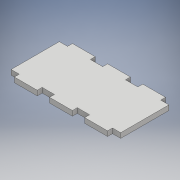
# Autodesk Inventor part: base4
Saved by Autodesk Inventor 2018 (Build 220112000, 112)
## iProperties
Created: 2020-03-10
Part Number: base4
Material: Genérico
Document SubType Name: Modeling
Designer: sala.ceri
Density: 1 g/cm^3
Appearance: Valor por defecto
Author: sala.ceri
Autodesk Inventor part; units mm, degrees
ref_plane "YZ Plane" through (0, 0, 0) normal (1, 0, 0) x (0, 1, 0)
ref_plane "XZ Plane" through (0, 0, 0) normal (0, 1, 0) x (-1, 0, 0)
ref_plane "XY Plane" through (0, 0, 0) normal (0, 0, 1) x (1, 0, 0)
sketch "Boceto1" plane through (0, 0, 0) normal (0, 1, 0) x (-1, 0, 0)
  circle A0 centre (28.5, 0) radius 1.5
  circle A1 centre (28.5, -8) radius 1.5
  circle A2 centre (28.5, 8) radius 1.5
  circle A3 centre (36.5, 0) radius 1.5
  circle A4 centre (20.5, 0) radius 1.5
  circle A5 centre (28.5, 0) radius 47.5
  line L0 (57, 33) -> (43, 33)
  line L1 (43, 33) -> (43, 30)
  line L2 (35.5, 30) -> (35.5, 33)
  line L3 (35.5, 33) -> (21.5, 33)
  line L4 (21.5, 33) -> (21.5, 30)
  line L5 (14, 30) -> (14, 33)
  line L6 (14, 33) -> (0, 33)
  line L7 (43, 30) -> (57, 30)
  line L8 (21.5, 30) -> (35.5, 30)
  line L9 (14, 30) -> (0, 30)
  line L10 (0, 30) -> (0, 33)
  line L11 (57, 33) -> (57, 30)
  line L12 (35.5, -30) -> (35.5, -33)
  line L13 (21.5, -30) -> (35.5, -30)
  line L14 (35.5, -33) -> (21.5, -33)
  line L15 (21.5, -33) -> (21.5, -30)
  line L16 (57, -33) -> (43, -33)
  line L17 (43, -33) -> (43, -30)
  line L18 (43, -30) -> (57, -30)
  line L19 (14, -30) -> (14, -33)
  line L20 (14, -30) -> (0, -30)
  line L21 (14, -33) -> (0, -33)
  line L22 (0, -30) -> (0, -33)
  line L23 (57, -33) -> (57, -30)
  constraints: 48 end point, 10 point on line, 6 centre point, 1 coincident, 1 vertical
extrude "Extrusión1" add sketch "Boceto1" along normal blind 3
sketch "Boceto2" plane through (-28.5, 0, 0) normal (0, -1, 0) x (1, 0, 0)
  circle A0 centre (0, 0) radius 3.5
  point P0 (28.5, 0)
  dimension "d23" = 7
  constraints: 1 centre point
  measures "d23" diameter of A0
extrude "Extrusión2" cut sketch "Boceto2" against normal blind 10
sketch "Boceto3" plane through (-28.5, 0, 0) normal (0, -1, 0) x (1, 0, 0)
  circle A0 centre (0, 0) radius 4.5
  point P0 (28.5, 0)
  dimension "d26" = 9
  constraints: 1 centre point
  measures "d26" diameter of A0
extrude "Extrusión3" cut sketch "Boceto3" against normal blind 10
sketch "Boceto4" plane through (-28.5, 0, 0) normal (0, -1, 0) x (1, 0, 0)
  circle A0 centre (0, 0) radius 4.5 projected
  arc A1 (-38.8091, 27.388) -> (38.8091, 27.388) centre (0, 0) ccw
  line L0 (-28.5, 30) -> (-28.5, 33) projected
  line L1 (-28.5, 30) -> (-28.5, 33)
  line L2 (-28.5, 33) -> (28.5, 33)
  line L3 (28.5, 33) -> (28.5, 30)
  line L4 (-14.5, 30) -> (-28.5, 30) projected
  line L5 (28.5, 30) -> (-28.5, 30)
  line L6 (-28.5, 33) -> (-31.5138, 33)
  line L7 (-31.5138, 33) -> (-31.5138, 30)
  line L8 (-31.5138, 30) -> (-28.5, 30)
  circle A2 centre (0, 0) radius 47.5 projected
  line L9 (38.8091, 27.388) -> (-38.8091, 27.388)
  point P0 (28.5, 0)
  constraints: 16 end point, 4 perpendicular, 4 point on circle, 2 horizontal, 1 centre point, 1 coincident, 1 collinear, 1 vertical
extrude "Extrusión4" cut sketch "Boceto4" against normal blind 10 contours L9 A1
sketch "Boceto5" plane through (0, 0, 0) normal (0, -1, 0) x (1, 0, 0)
  arc A0 (10.3091, 27.388) -> (-67.3091, 27.388) centre (-28.5, 0) ccw projected
  arc A1 (10.3091, 27.388) -> (-67.3091, 27.388) centre (-28.5, 0) ccw
  line L0 (-57, 19.347) -> (-43, 19.347)
  line L1 (0, 19.347) -> (-14, 19.347)
  line L2 (-14, 19.347) -> (-14, 16.347)
  line L3 (-21.5, 16.347) -> (-35.5, 16.347)
  line L4 (-43, 16.347) -> (-57, 16.347)
  line L5 (-57, 19.347) -> (-57, 16.347)
  line L6 (-43, 19.347) -> (-43, 16.347)
  line L7 (-35.5, 19.347) -> (-35.5, 16.347)
  line L8 (-21.5, 19.347) -> (-21.5, 16.347)
  line L9 (-14, 16.347) -> (0, 16.347)
  line L10 (0, 19.347) -> (0, 16.347)
  line L11 (-35.5, 19.347) -> (-21.5, 19.347)
  point P0 (0, 0)
  point P1 (-57, 30)
  point P2 (-21.5, 30)
  point P3 (0, 30)
  constraints: 24 end point, 6 point on line, 3 perpendicular, 2 parallel, 2 point on circle, 1 centre point, 1 coincident, 1 horizontal
extrude "Extrusión5" add sketch "Boceto5" against normal blind 3
sketch "Boceto6" plane through (0, 0, 0) normal (0, -1, 0) x (1, 0, 0)
  arc A0 (10.3091, 27.388) -> (-67.3091, 27.388) centre (-28.5, 0) ccw projected
  arc A1 (10.3091, 27.388) -> (-67.3091, 27.388) centre (-28.5, 0) ccw
  line L0 (-67.3091, 27.388) -> (10.3091, 27.388)
  point P0 (0, 0)
  constraints: 2 end point, 2 point on circle, 1 centre point, 1 coincident, 1 horizontal
extrude "Extrusión6" cut sketch "Boceto6" against normal blind 3
sketch "Boceto7" plane through (0, 0, 0) normal (0, -1, 0) x (1, 0, 0)
  line L0 (-57, 19.347) -> (-43, 19.347) projected
  line L1 (-57, 19.347) -> (-62, 19.347)
  line L2 (-62, 19.347) -> (-62, 16.347)
  line L3 (-62, 16.347) -> (5, 16.347)
  line L4 (5, 16.347) -> (5, 19.347)
  line L5 (5, 19.347) -> (-62, 19.347)
  point P0 (0, 0)
  dimension "d36" = 5
  dimension "d37" = 67
  constraints: 10 end point, 4 perpendicular, 1 horizontal, 1 point on line
  measures "d36" distance of L0.start L1.end
  measures "d37" distance of L2.end L3.end
extrude "Extrusión7" add sketch "Boceto7" along normal blind 29.5
sketch "Boceto8" plane through (0, -29.5, 0) normal (0, -1, 0) x (1, 0, 0)
  line L0 (-57, 19.347) -> (-43, 19.347) projected
  line L1 (-43, 16.347) -> (-57, 16.347) projected
  line L2 (-57, 19.347) -> (-57, 16.347)
  line L3 (-57, 16.347) -> (-43, 16.347)
  line L4 (-43, 19.347) -> (-43, 16.347) projected
  line L5 (-43, 16.347) -> (-43, 19.347)
  line L6 (-43, 19.347) -> (-57, 19.347)
  line L7 (-35.5, 19.347) -> (-21.5, 19.347) projected
  line L8 (-35.5, 19.347) -> (-35.5, 16.347)
  line L9 (-62, 16.347) -> (5, 16.347) projected
  line L10 (-21.5, 19.347) -> (-21.5, 16.347) projected
  line L11 (-35.5, 16.347) -> (-21.5, 16.347)
  line L12 (-21.5, 16.347) -> (-21.5, 19.347)
  line L13 (-21.5, 19.347) -> (-35.5, 19.347)
  line L14 (-14, 19.347) -> (0, 19.347) projected
  line L15 (-14, 19.347) -> (0, 19.347)
  line L16 (0, 19.347) -> (0, 16.347)
  line L17 (0, 16.347) -> (-14, 16.347)
  line L18 (-14, 16.347) -> (-14, 19.347) projected
  line L19 (-14, 16.347) -> (-14, 19.347)
  point P0 (0, 0)
  constraints: 24 end point, 6 perpendicular, 3 collinear, 3 point on line, 1 horizontal, 1 vertical
extrude "Extrusión8" add sketch "Boceto8" along normal blind 3
